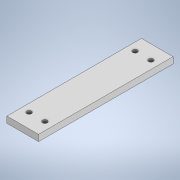
# Autodesk Inventor part: suporte estruzor 2
Saved by Autodesk Inventor 2022 (Build 260153000, 153)
## iProperties
Created: 2022-02-16
Part Number: suporte estruzor 2
Material: Genérico
Document SubType Name: Modeling
Designer: mathe
Density: 1 g/cm^3
Appearance: Padrão
Author: mathe
Autodesk Inventor part; units mm, degrees
ref_plane "YZ Plane" through (0, 0, 0) normal (1, 0, 0) x (0, 1, 0)
ref_plane "XZ Plane" through (0, 0, 0) normal (0, 1, 0) x (-1, 0, 0)
ref_plane "XY Plane" through (0, 0, 0) normal (0, 0, 1) x (1, 0, 0)
sketch "Esboço1" plane through (0, 0, 0) normal (0, 1, 0) x (-1, 0, 0)
  line L0 (0, 0) -> (20, 0)
  line L1 (20, 0) -> (20, -85)
  line L2 (20, -85) -> (0, -85)
  line L3 (0, -85) -> (0, 0)
  line L4 (0, -22) -> (20, -22)
  line L5 (20, -22) -> (20, -63)
  line L6 (20, -63) -> (0, -63)
  line L7 (0, -63) -> (0, -22)
  dimension "d0" = 20
  dimension "d1" = 85
  dimension "d2" = 20
  dimension "d3" = 41
  constraints: 16 end point, 4 parallel, 2 horizontal, 2 perpendicular
  measures "d0" distance of L1.end L2.end
  measures "d1" distance of L0.end L1.end
  measures "d2" distance of L5.end L6.end
  measures "d3" distance of L4.end L5.end
extrude "Extrusão1" add sketch "Esboço1" along normal blind 4 contours L0 L1 L4 L3 | L6 L1 L2 L3
extrude "Extrusão2" add sketch "Esboço1" along normal blind 4 contours L4 L1 L6 L3
sketch "Esboço2" plane through (0, 4, 0) normal (0, 1, 0) x (1, 0, 0)
  point P0 (0, 0)
  point P1 (-5, 9)
  point P2 (-15, 9)
  point P3 (-15, 76)
  point P4 (-5, 76)
hole "Furo1" at (-5, 4, -9) at (-15, 4, -9) at (-15, 4, -76) at (-5, 4, -76) direction (0, -1, 0) diameter 3 end through all
